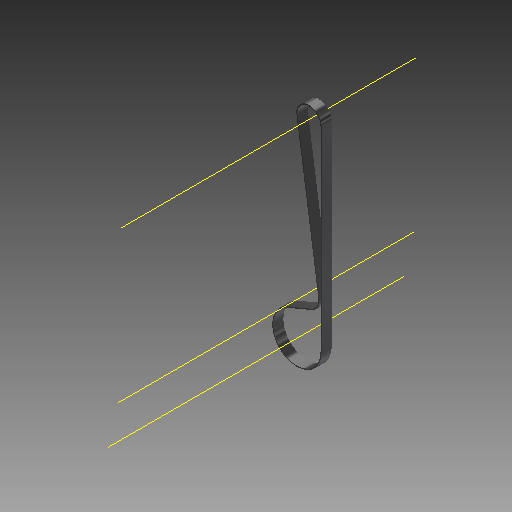
# Autodesk Inventor part: Synchronous Belt
Saved by Autodesk Inventor 2019.4 (Build 234330000, 330)
## iProperties
Created: 2020-02-16
Part Number: Synchronous Belt
Material: Rubber
Document SubType Name: Modeling
Designer: admin
Density: 1 g/cm^3
Appearance: Rubber - Black - Version 1.1
CustomPartVersion: 1
Author: admin
Autodesk Inventor part; units mm, degrees
sketch "Sketch Path" plane through (0, 0, 0) normal (0, 0, 1) x (1, 0, 0)
  arc A0 (101.3225, 289.5806) -> (77.5771, 287.8382) centre (89.3858, 289.5806) ccw
  arc A1 (68.1712, 118.521) -> (101.3225, 96.5244) centre (77.4493, 96.5244) ccw
  arc A2 (92.0249, 128.5823) -> (99.1946, 141.3229) centre (87.3858, 139.5806) ccw
  line L0 (99.1946, 141.3229) -> (77.5771, 287.8382)
  line L1 (101.3225, 289.5806) -> (101.3225, 96.5244)
  line L2 (68.1712, 118.521) -> (92.0249, 128.5823)
  constraints: 6 end point, 6 point on circle, 3 centre point
ref_plane "Cross Section Plane" through (77.5771, 287.8382, 0) normal (0.146, -0.9893, 0) x (0, 0, 1)
ref_plane "Work Plane2" through (89.3858, 289.5806, 0) normal (-1, 0, 0) x (0, 0, 1)
ref_plane "Work Plane3" through (77.4493, 96.5244, 0) normal (0.1334, 0.9911, 0) x (0, 0, 1)
ref_plane "Work Plane4" through (87.3858, 139.5806, 0) normal (0.4332, -0.9013, 0) x (0, 0, 1)
sketch "Cross Section" plane through (77.5771, 287.8382, 0) normal (0.146, -0.9893, 0) x (0, 0, 1)
  line L0 (-5, 0.5) -> (5, 0.5)
  line L1 (5, 0.5) -> (5, -0.5)
  line L2 (5, -0.5) -> (-5, -0.5)
  line L3 (-5, -0.5) -> (-5, 0.5)
  line L4 (-5, 0) -> (5, 0) construction
  point P0 (0, 0)
  point P1 (0, 0)
  dimension "d0" = 10
  dimension "d4" = 0.5
  dimension "d5" = 0.5
  constraints: 10 end point, 3 midpoint, 2 parallel, 1 coincident, 1 horizontal, 1 perpendicular, 1 other
  measures "d0" distance between parallel lines of L1 L3
  measures "d4" distance between parallel lines of L2 L4
  measures "d5" distance between parallel lines of L4 L0
sweep "Belt" add profiles "Cross Section" path "Sketch Path"
equation "\"d0\" = da_B"
equation "\"d4\" = da_a"
equation "\"d5\" = da_a2"
equation "\"da_B\" = 10"
equation "\"da_pb\" = 5"
equation "\"da_L\" = 525"
equation "\"da_a\" = 0.5"
equation "\"da_S\" = 2.65"
equation "\"da_Beta\" = 20deg"
equation "\"da_Ht\" = 1.2"
equation "\"da_H\" = 3.4"
equation "\"da_a2\" = 0.5"
body "Solid1"
